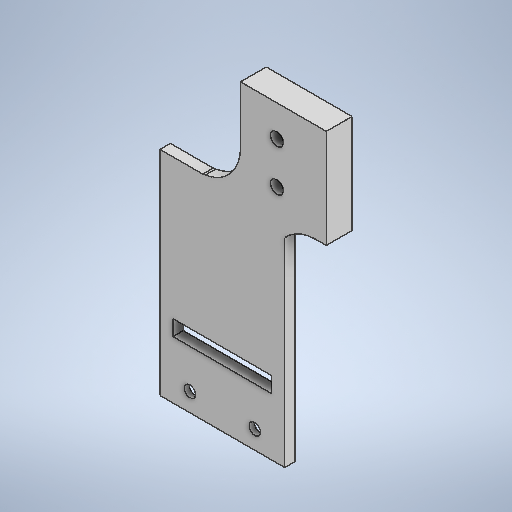
# Autodesk Inventor part: adapter_tof
Saved by Autodesk Inventor 2025 (Build 290162000, 162)
## iProperties
Created: 2025-11-03
Part Number: adapter_tof
Material: 一般
Document SubType Name: Modeling
Designer: sooo1
Density: 1 g/cm^3
Appearance: 既定
Author: sooo1
Autodesk Inventor part; units mm, degrees
ref_plane "YZ Plane" through (0, 0, 0) normal (1, 0, 0) x (0, 1, 0)
ref_plane "XZ Plane" through (0, 0, 0) normal (0, 1, 0) x (-1, 0, 0)
ref_plane "XY Plane" through (0, 0, 0) normal (0, 0, 1) x (1, 0, 0)
sketch "スケッチ1" plane through (0, 0, 0) normal (0, 0, 1) x (1, 0, 0)
  line L0 (-10, 30) -> (10, 30)
  line L1 (10, 30) -> (10, -30)
  line L2 (10, -30) -> (-10, -30)
  line L3 (-10, -30) -> (-10, 30)
  line L4 (-10, 30) -> (10, -30) construction
  line L5 (10, 30) -> (-10, -30) construction
  line L6 (10, 30) -> (20, 30)
  line L7 (20, 30) -> (20, 11)
  line L8 (20, 11) -> (10, 11)
  line L9 (10.5, 30) -> (10.5, 11) construction
  circle A0 centre (10.5, 24) radius 1.25
  circle A1 centre (10.5, 16) radius 1.25
  line L10 (3.5, 30) -> (3.5, 11)
  line L11 (3.5, 11) -> (-10, 11)
  circle A2 centre (-6.25, -26.44) radius 1.1
  line L12 (-10, -26.44) -> (10, -26.44) construction
  circle A3 centre (6.25, -26.44) radius 1.1
  line L13 (0, -30) -> (0, 30) construction
  line L14 (-9.5, -15.94) -> (9.5, -15.94)
  line L15 (9.5, -15.94) -> (9.5, -18.94)
  line L16 (9.5, -18.94) -> (-9.5, -18.94)
  line L17 (-9.5, -18.94) -> (-9.5, -15.94)
  line L18 (-9.5, -15.94) -> (9.5, -18.94) construction
  line L19 (9.5, -15.94) -> (-9.5, -18.94) construction
  line L20 (10, 11) -> (3.5, 11)
  circle A4 centre (6.25, -26.44) radius 2.5
  circle A5 centre (-6.25, -26.44) radius 2.5
  line L21 (10, -30) -> (12, -30)
  line L22 (12, -30) -> (12, 11)
  line L23 (-10, 11) -> (-12, 11)
  line L24 (-12, 11) -> (-12, -30)
  line L25 (-12, -30) -> (-10, -30)
  point P0 (0, 0)
  point P1 (0, -17.44)
  dimension "d0" = 60
  dimension "d1" = 20
  dimension "d2" = 2.5
  dimension "d3" = 8
  dimension "d4" = 5
  dimension "d5" = 10.5
  dimension "d6" = 19
  dimension "d7" = 10
  dimension "d8" = 7
  dimension "d9" = 2.2
  dimension "d10" = 2.2
  dimension "d11" = 12.5
  dimension "d12" = 6.25
  dimension "d13" = 3.56
  dimension "d14" = 3
  dimension "d15" = 19
  dimension "d16" = 9
  dimension "d22" = 5
  dimension "d23" = 5
  dimension "d27" = 2
  dimension "d28" = 2
  constraints: 52 end point, 15 point on line, 12 perpendicular, 6 centre point, 6 midpoint, 4 horizontal, 4 parallel, 2 coincident, 1 collinear, 1 equal radius, 1 vertical
  measures "d0" distance of L2.end L0.start
  measures "d1" distance of L0.start L0.end
  measures "d2" diameter of A0
  measures "d3" distance of A1.centre A0.centre
  measures "d4" distance from line of L8 A1.centre
  measures "d5" distance from line of point (0, 0) L9
  measures "d6" distance of L6.end L7.end
  measures "d7" distance between parallel lines of L1 L7
  measures "d8" distance between parallel lines of L10 L9
  measures "d9" diameter of A2
  measures "d10" diameter of A3
  measures "d11" distance of A3.centre A2.centre
  measures "d12" distance from line of L13 A2.centre
  measures "d13" distance between parallel lines of L2 L12
  measures "d14" distance of L16.end L14.start
  measures "d15" distance of L14.start L14.end
  measures "d16" distance from line of L12 point (0, -17.44)
  measures "d22" diameter of A4
  measures "d23" diameter of A5
  measures "d27" distance between parallel lines of L1 L22
  measures "d28" distance between parallel lines of L3 L24
extrude "押し出し1" add sketch "スケッチ1" along normal blind 2 contours L0 L1 A0 A1 L20 L10 | L11 L20 L1 L2 L3 | L6 L7 L8 L1 A1 A0 | A4 | A5
extrude "押し出し2" add sketch "スケッチ1" against normal blind 2.95 contours L0 L1 A0 A1 L20 L10 | L6 L7 L8 L1 A1 A0
fillet "フィレット1" radius 8 2 edges at (10, 11, 1) (3.5, 11, 1)
extrude "押し出し3" cut sketch "スケッチ1" along normal blind 1 contours A4 | A5
fillet "フィレット2" radius 8 1 edges at (-10, 11, 1)
extrude "押し出し4" add sketch "スケッチ1" along normal up to surface (2 mm away) contours L11 L20 L1 L2 L3 | L3 L25 L24 L23 | L8 L22 L21 L1
